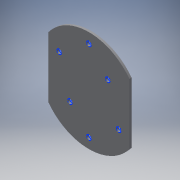
# Autodesk Inventor part: PCB_PLACEHOLDER
Saved by Autodesk Inventor 2016 (Build 200138000, 138)
## iProperties
Created: 2016-09-17
Part Number: PCB_PLACEHOLDER
Material: Generic
Document SubType Name: Modeling
Designer: benja
Density: 1 g/cm^3
Appearance: Default
Author: benja
Autodesk Inventor part; units mm, degrees
ref_plane "YZ Plane" through (0, 0, 0) normal (1, 0, 0) x (0, 1, 0)
ref_plane "XZ Plane" through (0, 0, 0) normal (0, 1, 0) x (-1, 0, 0)
ref_plane "XY Plane" through (0, 0, 0) normal (0, 0, 1) x (1, 0, 0)
sketch "Sketch1" plane through (0, 0, 0) normal (0, 0, 1) x (1, 0, 0)
  circle A0 centre (0, 0) radius 37.5
  line L0 (-30, 22.5) -> (-30, -22.5)
  line L1 (30, 22.5) -> (30, -22.5)
  dimension "d0" = 75
  dimension "d20" = 45
  constraints: 4 end point, 4 point on circle, 2 parallel, 1 centre point, 1 coincident, 1 vertical
  measures "d0" diameter of A0
  measures "d20" distance of L0.start L0.end
extrude "Extrusion1" add sketch "Sketch1" along normal blind 1.5875 contours L1 A0 L0
sketch "Sketch2" plane through (0, 0, 1.5875) normal (0, 0, 1) x (1, 0, 0)
  circle A0 centre (-14, -14) radius 1.75
  line L0 (30, -22.5) -> (30, 22.5) projected
  line L1 (-30, 22.5) -> (-30, -22.5) projected
  point P0 (0, 0)
  point P1 (22, -14)
  point P2 (14, 14)
  point P3 (-22, 14)
  point P4 (0, -25)
  point P5 (0, 30)
  dimension "d11" = 8
  dimension "d15" = 16
  dimension "d21" = 16
  dimension "d24" = 8
  dimension "d26" = 28
  dimension "d27" = 28
  dimension "d28" = 14
  dimension "d29" = 14
  dimension "d30" = 25
  dimension "d31" = 30
  constraints: 2 vertical alignment, 1 centre point, 1 coincident
  measures "d11" distance from line of L0 point (22, -14)
  measures "d15" distance from line of L1 A0.centre
  measures "d21" distance from line of L0 point (14, 14)
  measures "d24" distance from line of L1 point (-22, 14)
  measures "d26" vertical distance of A0.centre point (-22, 14)
  measures "d27" vertical distance of point (22, -14) point (14, 14)
  measures "d28" vertical distance of point (0, 0) point (22, -14)
  measures "d29" horizontal distance of point (0, 0) point (-14, -14)
  measures "d30" distance of point (0, 0) point (0, -25)
  measures "d31" distance of point (0, 0) point (0, 30)
hole "Hole1" at (22, -14, 1.5875) at (14, 14, 1.5875) at (-14, -14, 1.5875) at (-22, 14, 1.5875) at (0, -25, 1.5875) at (0, 30, 1.5875) direction (0, 0, -1) diameter 3.5 end through all
equation "\"d15\" = d21"
equation "\"d24\" = d11"
equation "\"d27\" = d26"
equation "\"d28\" = 0.5 * d27"
equation "\"d29\" = 0.5 * d26"
body "Solid1"
